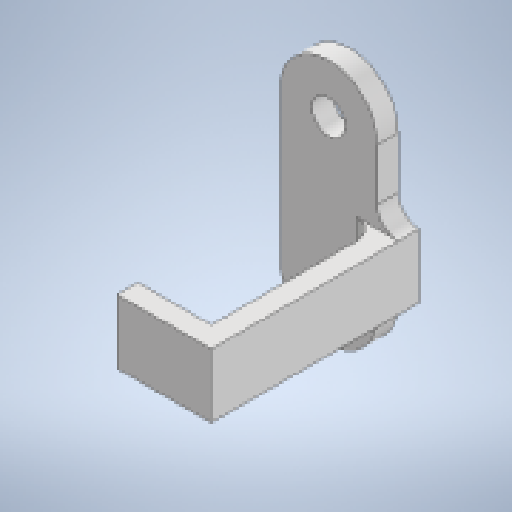
# Autodesk Inventor part: j2 endstop blocker
Saved by Autodesk Inventor 2025 (Build 290162000, 162)
## iProperties
Created: 2025-08-04
Part Number: j2 endstop blocker
Material: 一般
Document SubType Name: Modeling
Designer: gavin
Density: 1 g/cm^3
Appearance: 預設
Author: gavin
## iProperties of the stored document j2 endstop blocker_3D 列印.ipt
Created: 2025-08-04
Part Number: j2 endstop blocker_3D 列印
Material: 一般
Document SubType Name: Modeling
Designer: gavin
Density: 1 g/cm^3
Appearance: 預設
Author: gavin
Autodesk Inventor part; units mm, degrees
sketch "草圖1" plane through (0, 0, 0) normal (0, 0, 1) x (1, 0, 0)
  circle A0 centre (48.975, 7.075) radius 2.165 projected
  circle A1 centre (48.975, -7.075) radius 2.165 projected
  circle A2 centre (0, 0) radius 37.575 projected
  line L0 (40.0902, 13.075) -> (66.575, 13.075) projected
  arc A3 (36.4101, 15.5076) -> (40.0902, 13.075) centre (40.0902, 17.075) ccw projected
  arc A4 (36.4101, 15.5076) -> (37.3527, -13.075) centre (0, 0) ccw projected
  line L1 (66.575, -13.075) -> (37.3527, -13.075) projected
  line L2 (66.575, 13.075) -> (66.575, -13.075) projected
  line L3 (52.955, -6) -> (43.155, -6) construction
  line L4 (52.955, -6) -> (52.955, 0.1) construction
  line L5 (43.155, 0.1) -> (52.955, 0.1) construction
  line L6 (43.155, -6) -> (43.155, 0.1) construction
  arc A5 (44.4356, -6) -> (53.64, -7.075) centre (48.975, -7.075) ccw
  arc A6 (53.64, 7.075) -> (44.31, 7.075) centre (48.975, 7.075) ccw
  line L7 (53.64, -7.075) -> (53.64, 7.075)
  line L8 (44.31, -7.075) -> (44.31, 7.075)
  circle A7 centre (48.975, -7.075) radius 1.6
  circle A8 centre (48.975, 7.075) radius 1.6
  point P0 (0, 0)
  dimension "d0" = 2.5
  dimension "d1" = 2.5
  dimension "d14" = 3.2
  dimension "d15" = 3.2
  constraints: 5 point on circle, 4 centre point, 4 end point, 2 coincident, 1 parallel, 1 point on line, 1 tangent, 1 vertical
  measures "d0" radial gap between concentric circles of A1 A5
  measures "d1" radial gap between concentric circles of A0 A6
  measures "d14" diameter of A7
  measures "d15" diameter of A8
extrude "擠出1" add sketch "草圖1" along normal blind 2 contours A0 | A1 | L8 A6 L7 A5
ref_plane "工作平面1" through (41.575, -6, 34.5) normal (0, -1, 0) x (1, 0, 0)
sketch "草圖2" plane through (41.575, -6, 34.5) normal (0, -1, 0) x (1, 0, 0)
  line L0 (0, 0) -> (0, -28) projected
  line L1 (0, -28) -> (1.58, -28) projected
  line L2 (1.58, -24) -> (1.58, -28) projected
  line L3 (1.58, -24) -> (11.38, -24) projected
  line L4 (11.38, -24) -> (11.38, -20) projected
  line L5 (11.38, -20) -> (3.42, -20) projected
  line L6 (3.42, -20) -> (3.42, -15.06) projected
  line L7 (3.42, -15.06) -> (11.38, -15.06) projected
  line L8 (11.38, -15.06) -> (11.38, -11.06) projected
  line L9 (11.38, -11.06) -> (1.58, -11.06) projected
  line L10 (1.58, 0) -> (1.58, -11.06) projected
  line L11 (0, 0) -> (1.58, 0) projected
  line L12 (2.735, -34.5) -> (12.065, -34.5) projected
  line L13 (12.065, -34.5) -> (12.065, -32.5) projected
  line L14 (2.735, -32.5) -> (12.065, -32.5) projected
  line L15 (2.735, -34.5) -> (2.735, -32.5) projected
  line L16 (5.065, -16.64) -> (12.065, -16.64)
  line L17 (12.065, -16.64) -> (12.065, -32.5)
  line L18 (12.065, -32.5) -> (12.065, -32.5)
  line L19 (12.065, -34.5) -> (14.065, -34.5)
  line L20 (14.065, -34.5) -> (14.065, -14.64)
  line L21 (14.065, -14.64) -> (5.065, -14.64)
  line L22 (5.065, -14.64) -> (5.065, -16.64)
  point P0 (-41.575, -34.5)
  dimension "d4" = 2
  dimension "d5" = 2
  dimension "d9" = 7
  dimension "d17" = 19.86
  constraints: 14 end point, 5 perpendicular, 2 horizontal, 1 point on line
  measures "d4" distance between parallel lines of L16 L21
  measures "d5" distance between parallel lines of L17 L20
  measures "d9" distance of L16.start L16.end
  measures "d17" distance of L19.end L20.end
ref_plane "工作平面2" through (43.155, 0.1, 10.5) normal (0, 1, 0) x (0, 0, 1)
ref_plane "工作平面3" through (43.155, 0.1, 10.5) normal (0, 1, 0) x (0, 0, 1)
extrude "擠出2" add sketch "草圖2" against normal up to surface (6.1 mm away) contours L21 L20 L19 L13 L17 L16 L22 L7 L8 | L8 L7 L22 L21
fillet "圓角2" radius 2 3 edges at (53.64, -6, 1) (53.64, -2.95, 2) (53.64, 0.1, 1)
